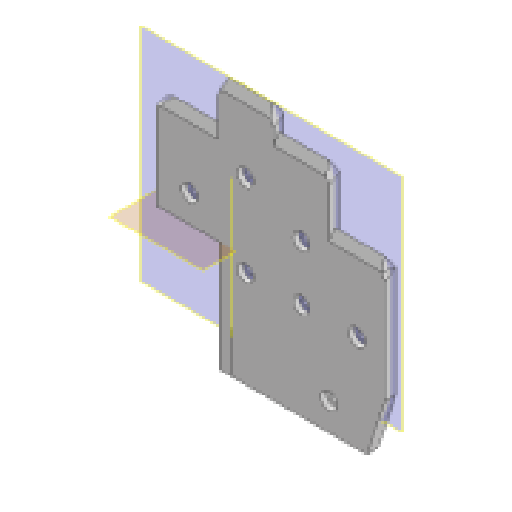
# Autodesk Inventor part: Palm
Saved by Autodesk Inventor 2025 (Build 290162010, 162A)
## iProperties
Created: 2024-12-07
Part Number: Palm
Material: Generic
Document SubType Name: Modeling
Designer: alexa
Density: 1 g/cm^3
Appearance: Default
Author: alexa
Autodesk Inventor part; units mm, degrees
ref_plane "YZ Plane" through (0, 0, 0) normal (1, 0, 0) x (0, 1, 0)
ref_plane "XZ Plane" through (0, 0, 0) normal (0, 1, 0) x (-1, 0, 0)
ref_plane "XY Plane" through (0, 0, 0) normal (0, 0, 1) x (1, 0, 0)
sketch "Sketch1" plane through (0, 0, 0) normal (0, 0, 1) x (1, 0, 0)
  line L0 (36.0199, -42.7926) -> (-34.4552, -42.7926)
  line L1 (-34.4552, -42.7926) -> (-34.4552, -11.0426)
  line L2 (-34.4552, -11.0426) -> (-73.3934, -11.0426)
  line L3 (-73.3934, -11.0426) -> (-73.3934, 18.523)
  line L4 (-73.3934, 18.523) -> (-69.4155, 29.59)
  line L5 (-69.4155, 29.59) -> (-40.9421, 29.59)
  line L6 (-40.9421, 29.59) -> (-40.9421, 49.91)
  line L7 (-40.9421, 49.91) -> (-15.2881, 49.91)
  line L8 (-15.2881, 49.91) -> (-15.2881, 39.75)
  line L9 (-15.2881, 39.75) -> (10.3659, 39.75)
  line L10 (10.3659, 39.75) -> (10.3659, 14.35)
  line L11 (10.3659, 14.35) -> (36.0199, 14.35)
  line L12 (36.0199, 14.35) -> (36.0199, -42.7926)
  point P0 (0, 0)
  dimension "d1" = 31.75
  dimension "d2" = 38.9382
  dimension "d3" = 29.5656
  dimension "d4" = 11.7602
  dimension "d5" = 19.77
  dimension "d6" = 28.4734
  dimension "d7" = 20.32
  dimension "d8" = 25.654
  dimension "d9" = 25.654
  dimension "d10" = 25.654
  dimension "d11" = 10.16
  dimension "d12" = 25.4
  constraints: 26 end point, 6 perpendicular, 3 horizontal, 3 vertical
  measures "d1" distance of L0.end L1.end
  measures "d2" distance of L1.end L2.end
  measures "d3" distance of L2.end L3.end
  measures "d4" distance of L3.end L4.end
  measures "d5" angle of L4 L1
  measures "d6" distance of L4.end L5.end
  measures "d7" distance of L5.end L6.end
  measures "d8" distance of L6.end L7.end
  measures "d9" distance of L8.end L9.end
  measures "d10" distance of L10.end L11.end
  measures "d11" distance of L7.end L8.end
  measures "d12" distance of L9.end L10.end
extrude "Extrusion1" add sketch "Sketch1" along normal blind 5.08
sketch "Sketch3" plane through (-34.4552, -42.7926, 0) normal (0, -1, 0) x (1, 0, 0)
  line L0 (0.0059, 0) -> (-3.82, 3.4008) projected
  line L1 (0, 0) -> (0, 5.08) projected
  line L2 (0, 0) -> (0, 5.08)
  line L3 (19.167, 5.08) -> (-6.487, 5.08) projected
  line L4 (0, 5.08) -> (0, 0)
  line L5 (0, 5.08) -> (-5.7091, 5.08)
  line L6 (-5.7091, 5.08) -> (0, 0)
  point P0 (34.4552, 0)
  point P1 (-5.7091, 5.08)
  point P2 (0, 0.0053)
  point P3 (-5.7091, 5.08)
  constraints: 8 end point, 2 point on line, 1 collinear, 1 perpendicular, 1 vertical
extrude "Extrusion3" add sketch "Sketch3" against normal blind 57.15
sketch "Sketch4" plane through (-73.3934, -11.0426, 0) normal (0, -1, 0) x (1, 0, 0)
  line L0 (17.1894, 19.3376) -> (-10.63, -11.9592) projected
  line L1 (0, 5.08) -> (38.9382, 5.08) projected
  line L2 (0, -0.0005) -> (0, 5.08)
  line L3 (0, 5.08) -> (4.516, 5.08)
  line L4 (4.516, 5.08) -> (0, -0.0005)
  point P0 (73.3934, 0)
  point P1 (33.2291, 5.08)
  point P2 (4.516, 5.08)
  constraints: 6 end point, 2 perpendicular, 2 point on line, 1 collinear
sketch "Sketch5" plane through (-40.9421, 29.59, 0) normal (-1, 0, 0) x (0, 0, 1)
  line L0 (2.54, 4.4068) -> (-12.7, -21.9897) projected
  line L1 (5.08, 0) -> (5.08, -11.067) projected
  line L2 (5.08, 0) -> (2.54, 4.4068)
  line L3 (2.54, 4.4068) -> (-0.0043, 0)
  line L4 (0, 0) -> (0, -11.067) projected
  line L5 (0, 0) -> (5.08, 0)
  line L6 (2.54, 4.4068) -> (0, 0)
  line L7 (0, 0) -> (5.08, 0)
  line L8 (5.08, 0) -> (2.54, 4.4068)
  point P0 (0, -29.59)
  constraints: 12 end point, 1 collinear, 1 horizontal, 1 perpendicular, 1 point on line
extrude "Extrusion4" add sketch "Sketch5" along normal up to surface surface through (-69.4155, 29.59, 0) normal (-0.941058, 0.3382452, 0)
extrude "Extrusion5" cut sketch "Sketch4" against normal blind 66.675
sketch "Sketch6" plane through (-40.9421, 29.59, 0) normal (0, 0.4993725, -0.8663874) x (-1, 0, 0)
  line L0 (25.654, 0.0178) -> (28.4749, 0.0064) projected
  line L1 (22.987, -32.5297) -> (22.987, 6.2121) projected
  line L2 (0, 5.0864) -> (26.8895, 5.0864) projected
  line L3 (22.987, 5.0864) -> (29.2176, 0.0225)
  line L4 (32.4508, -9.5873) -> (28.2515, 2.894) projected
  line L5 (29.2176, 0.0225) -> (22.987, 0.0225)
  line L6 (22.987, 0.0225) -> (22.987, 5.0864)
  line L7 (22.987, 5.0864) -> (26.8895, 5.0864)
  line L8 (26.8895, 5.0864) -> (28.2515, 2.894) projected
  line L9 (26.8895, 5.0864) -> (28.2515, 2.894)
  line L10 (28.2515, 2.894) -> (29.2176, 0.0225)
  point P0 (-40.9421, -25.6364)
  constraints: 12 end point, 4 point on line, 3 collinear, 1 horizontal, 1 perpendicular
extrude "Extrusion6" cut sketch "Sketch6" against normal blind 11.1125 contours L2 L8 L4 L3
sketch "Sketch7" plane through (-40.9421, 49.91, 0) normal (-1, 0, 0) x (0, 0, 1)
  line L0 (-12.7, -21.9897) -> (2.54, 4.4068) projected
  line L1 (0, 0) -> (5.08, 0) projected
  line L2 (2.54, 4.4068) -> (5.08, 0)
  line L3 (5.08, 0) -> (0, 0)
  line L4 (0, 0) -> (2.54, 4.4068)
  point P0 (0, -49.91)
  constraints: 6 end point, 1 collinear
extrude "Extrusion7" add sketch "Sketch7" against normal up to surface (25.654 mm away)
sketch "Sketch8" plane through (10.3659, 14.35, 0) normal (1, 0, 0) x (0, 0, -1)
  line L0 (12.7, -21.9897) -> (-2.54, 4.4068) projected
  line L1 (0, 0) -> (-5.08, 0) projected
  line L2 (-2.54, 4.4068) -> (-5.08, 0)
  line L3 (-5.08, 0) -> (0, 0.0074)
  line L4 (0, -25.3926) -> (0, 4.1741) projected
  line L5 (0, 0.0074) -> (-2.54, 4.4068)
  point P0 (0, -14.35)
  constraints: 6 end point, 2 point on line
extrude "Extrusion8" add sketch "Sketch8" along normal up to surface (25.654 mm away) contours L3 L2 L0
sketch "Sketch9" plane through (36.0199, 14.3574, 0) normal (0, 0.5, -0.8660254) x (-1, 0, 0)
  line L0 (2.667, -32.5754) -> (2.667, 6.1663) projected
  line L1 (2.54, 0) -> (0, 0) projected
  line L2 (0, 0) -> (2.667, 5.08)
  line L3 (25.654, 5.08) -> (0, 5.08) projected
  line L4 (0, 5.08) -> (0, 0) projected
  line L5 (2.667, 5.08) -> (0, 5.08)
  line L6 (0, 5.08) -> (0, 0)
  point P0 (36.0199, -12.4339)
  constraints: 6 end point, 2 perpendicular, 2 point on line
extrude "Extrusion9" cut sketch "Sketch9" against normal blind 14.2875
sketch "Sketch10" plane through (-15.2881, 39.75, 5.08) normal (1, 0, 0) x (0, 0, -1)
  line L0 (2.54, 4.4068) -> (17.78, -21.9897) projected
  line L1 (0, -25.4) -> (0, 0) projected
  line L2 (2.54, 4.4068) -> (0, 0)
  line L3 (0, 0) -> (5.08, 0)
  line L4 (5.08, 10.16) -> (5.08, -10.16) projected
  line L5 (5.08, 0) -> (0, 0)
  line L6 (5.08, 0) -> (2.54, 4.4068)
  point P0 (5.08, -39.75)
  constraints: 8 end point, 1 collinear, 1 midpoint
extrude "Extrusion10" add sketch "Sketch10" along normal up to surface (25.654 mm away) contours L6 L3 L2
sketch "Sketch11" plane through (10.3659, 39.75, 0) normal (0, 0.4993725, -0.8663874) x (-1, 0, 0)
  line L0 (2.667, -32.5297) -> (2.667, 6.2121) projected
  line L1 (2.54, 0.0178) -> (0, 0.0178) projected
  line L2 (0, -21.9999) -> (0, 0) projected
  line L3 (0, 0) -> (2.667, 5.0864)
  line L4 (25.654, 5.0864) -> (0, 5.0864) projected
  line L5 (2.667, 5.0864) -> (0, 5.0864)
  line L6 (0, 5.0864) -> (0, 0)
  point P0 (10.3659, -34.4389)
  constraints: 6 end point, 2 point on line, 1 collinear, 1 perpendicular
extrude "Extrusion11" cut sketch "Sketch11" against normal blind 14.2875
sketch "Sketch12" plane through (-15.2881, 49.91, 0) normal (0, 0.4993725, -0.8663874) x (-1, 0, 0)
  line L0 (2.667, -32.5297) -> (2.667, 6.2121) projected
  line L1 (2.54, 0.0178) -> (0, 0.0178) projected
  line L2 (22.987, -32.5297) -> (22.987, 6.2121) projected
  line L3 (23.114, 0.0178) -> (25.654, 0.0178) projected
  line L4 (0, 0.0178) -> (2.667, 5.0864)
  line L5 (25.654, 5.0864) -> (0, 5.0864) projected
  line L6 (2.667, 5.0864) -> (0, 5.0864)
  line L7 (0, 5.0864) -> (0, 0.0178)
  line L8 (25.654, 0.0178) -> (22.987, 5.0864)
  line L9 (22.987, 5.0864) -> (25.654, 5.0864)
  line L10 (25.654, 5.0864) -> (25.654, 0.0178)
  point P0 (-15.2881, -43.2414)
  point P1 (25.654, 5.0864)
  point P2 (22.987, 5.0864)
  constraints: 12 end point, 5 point on line, 2 perpendicular, 1 collinear
extrude "Extrusion12" cut sketch "Sketch12" against normal blind 30.1625
ref_plane "Work Plane1" through (-63.2227, -11.0426, -4.7625) normal (0, 1, 0) x (0, 0, -1)
sketch "Sketch13" plane through (0, 0, 5.08) normal (0, 0, 1) x (1, 0, 0)
  line L0 (-15.2881, 49.9174) -> (-15.2881, -36.4426) projected
  line L1 (-40.9421, 29.5974) -> (-40.9421, -36.4426) projected
  line L2 (-15.2881, 49.9174) -> (-15.2881, -36.4426) projected
  line L3 (10.3659, 39.7574) -> (10.3659, -36.4426) projected
  line L4 (36.0199, 14.3574) -> (36.0199, -36.4426) projected
  circle A0 centre (-28.1151, -17.3926) radius 1.778
  circle A1 centre (-2.4611, -17.3926) radius 1.778
  circle A2 centre (23.1929, -17.3926) radius 1.778
  line L5 (36.0199, -42.7926) -> (-40.1643, -42.7926) projected
  circle A3 centre (-28.1151, 20.7074) radius 1.778
  circle A4 centre (-2.4611, 8.0074) radius 1.778
  circle A5 centre (-53.7691, 1.6574) radius 1.778
  line L6 (-66.5961, 29.5974) -> (-66.5961, 14.3574) projected
  line L7 (-73.393, -11.0426) -> (-34.4552, -11.0426) projected
  point P0 (0, 0)
  dimension "d38" = 3.556
  dimension "d39" = 3.556
  dimension "d40" = 3.556
  dimension "d41" = 12.827
  dimension "d42" = 12.827
  dimension "d43" = 12.827
  dimension "d44" = 25.4
  dimension "d45" = 3.556
  dimension "d46" = 3.556
  dimension "d47" = 38.1
  dimension "d48" = 25.4
  dimension "d53" = 3.556
  dimension "d54" = 12.827
  dimension "d55" = 12.7
  constraints: 6 centre point, 2 horizontal alignment, 2 vertical alignment, 1 other
  measures "d38" diameter of A0
  measures "d39" diameter of A1
  measures "d40" diameter of A2
  measures "d41" distance from line of L0 A0.centre
  measures "d42" distance from line of L0 A1.centre
  measures "d43" distance from line of L3 A2.centre
  measures "d44" distance from line of L5 A0.centre
  measures "d45" diameter of A3
  measures "d46" diameter of A4
  measures "d47" distance of A3.centre A0.centre
  measures "d48" distance of A4.centre A1.centre
  measures "d53" diameter of A5
  measures "d54" distance from line of L1 A5.centre
extrude "Extrusion15" cut sketch "Sketch13" along normal blind 127 and the other way blind 127
ref_plane "Work Plane2" through (0, 0, 2.54) normal (0, 0, -1) x (-1, 0, 0)
sketch "Sketch17" plane through (0, 0, 2.54) normal (0, 0, -1) x (-1, 0, 0)
  circle A0 centre (28.1151, 20.7074) radius 1.778 projected
  circle A1 centre (28.1151, 20.7074) radius 3.81
  circle A2 centre (2.4611, 8.0074) radius 1.778 projected
  circle A3 centre (2.4611, 8.0074) radius 3.81
  circle A4 centre (2.4611, -17.3926) radius 1.778 projected
  circle A5 centre (2.4611, -17.3926) radius 3.81
  circle A6 centre (-23.1929, -17.3926) radius 1.778 projected
  circle A7 centre (-23.1929, -17.3926) radius 3.81
  circle A8 centre (28.1151, -17.3926) radius 1.778 projected
  circle A9 centre (28.1151, -17.3926) radius 3.81
  circle A10 centre (53.7691, 1.6574) radius 1.778 projected
  circle A11 centre (53.7691, 1.6574) radius 3.81
  point P0 (0, 0)
  dimension "d61" = 7.62
  dimension "d62" = 7.62
  dimension "d63" = 7.62
  dimension "d64" = 7.62
  dimension "d65" = 7.62
  dimension "d66" = 7.62
  constraints: 6 centre point, 6 coincident
  measures "d61" diameter of A11
  measures "d62" diameter of A1
  measures "d63" diameter of A3
  measures "d64" diameter of A9
  measures "d65" diameter of A5
  measures "d66" diameter of A7
extrude "Extrusion16" cut sketch "Sketch17" against normal blind 127 contours A1 | A3 | A4 | A5 | A6 | A7 | A9 | A11
sketch "Sketch18" plane through (0, 0, 5.08) normal (0, 0, 1) x (1, 0, 0)
  line L0 (-73.393, 14.3574) -> (-56.204, 14.3574) projected
  line L1 (-56.204, 14.3574) -> (-34.4493, 14.3574) projected
  line L2 (-34.4493, -36.4426) -> (-34.4493, 14.3574) projected
  line L3 (-68.8774, -11.0426) -> (-73.393, -11.0426) projected
  line L4 (-73.393, -11.0426) -> (-73.393, 18.5242) projected
  line L5 (-73.393, 14.3574) -> (-34.4552, 14.3574)
  line L6 (-34.4552, 14.3574) -> (-34.4552, -11.0426)
  line L7 (-73.393, -11.0426) -> (-73.393, 14.3574)
  line L8 (-73.393, -11.0426) -> (-34.4552, -11.0426) projected
  line L9 (-73.393, -11.0426) -> (-34.4552, -11.0426)
  point P0 (0, 0)
  constraints: 8 end point, 2 horizontal, 1 parallel, 1 perpendicular
extrude "Extrusion18" cut sketch "Sketch18" against normal blind 127
ref_plane "Work Plane3" through (-33.8301, -42.7926, 0) normal (1, 0, 0) x (0, 0, -1)
sketch "Sketch20" plane through (-33.8301, -42.7926, 0) normal (1, 0, 0) x (0, 0, -1)
  line L0 (-19.3376, 31.75) -> (0, 57.15) projected
  line L1 (-5.08, 57.15) -> (-5.08, 50.4774)
  line L2 (-5.08, 50.4774) -> (0, 57.15)
  line L3 (0, 0) -> (0, 57.1426) projected
  line L4 (0, 57.1426) -> (-5.08, 57.15)
  line L5 (-5.08, 50.4774) -> (-5.08, 31.75)
  line L6 (-5.08, 31.75) -> (-19.3376, 31.75)
  point P0 (0, 42.7926)
  point P1 (-0.0056, 57.1426)
  constraints: 10 end point, 1 perpendicular, 1 point on line, 1 vertical
extrude "Extrusion20" add sketch "Sketch20" against normal up to surface contours L1 L4 L0 surface through (-68.8774, -11.0426, 5.08) normal (0.7474093, 0, -0.6643638)
sketch "Sketch21" plane through (0, 0, 5.08) normal (0, 0, 1) x (1, 0, 0)
  line L0 (27.7649, -61.8426) -> (36.0199, -36.4426) projected
  line L1 (36.0199, -42.7926) -> (36.0199, 14.35) projected
  line L2 (36.0199, -36.4426) -> (36.0199, -42.7926)
  line L3 (36.0199, -42.7926) -> (33.9561, -42.7926)
  point P0 (0, 0)
  constraints: 4 end point, 1 collinear, 1 perpendicular, 1 point on line
extrude "Extrusion21" cut sketch "Sketch21" against normal blind 23.495
sketch "Sketch22" plane through (0, 0, 5.08) normal (0, 0, 1) x (1, 0, 0)
  line L0 (27.7649, -61.8426) -> (-34.4493, -61.8426) projected
  line L1 (27.7649, -61.8426) -> (36.0199, -36.4426) projected
  line L2 (-38.2751, -36.4426) -> (-38.2751, -61.8426) projected
  line L3 (-34.4493, -61.8426) -> (-48.4634, -61.8426) projected
  line L4 (33.9561, -42.7926) -> (-40.1643, -42.7926) projected
  line L5 (-34.4552, -42.7926) -> (-34.4552, -42.7926) projected
  line L6 (-34.4552, -42.7926) -> (-34.4493, -61.8426)
  point P0 (0, 0)
  point P1 (-38.2751, -42.7926)
  point P2 (-34.4552, 14.3574)
  constraints: 2 end point, 1 vertical alignment
extrude "Extrusion22" add sketch "Sketch22" against normal blind 5.08 contours L0 L6 L4 L1
sketch "Sketch23" plane through (-40.1643, -42.7926, 5.08) normal (0, -1, 0) x (1, 0, 0)
  line L0 (5.7091, -5.08) -> (5.7091, 0) projected
  line L1 (5.7091, 0) -> (0, 0) projected
  line L2 (0, 0) -> (5.7091, -5.08) projected
  point P0 (40.1643, -5.08)
extrude "Extrusion23" add sketch "Sketch23" along normal up to surface (19.05 mm away)
sketch "Sketch24" plane through (0, 0, 5.08) normal (0, 0, 1) x (1, 0, 0)
  line L0 (1.3489, -61.8426) -> (-6.2711, -61.8426) projected
  line L1 (27.0029, -61.8426) -> (19.3829, -61.8426) projected
  circle A0 centre (10.3659, -49.1426) radius 1.778
  line L2 (-34.4493, -61.8426) -> (27.7649, -61.8426) projected
  point P0 (0, 0)
  dimension "d84" = 3.556
  dimension "d85" = 18.034
  dimension "d86" = 9.017
  dimension "d87" = 12.7
  constraints: 1 centre point
  measures "d84" diameter of A0
  measures "d85" distance of L1.end L0.start
  measures "d86" horizontal distance of A0.centre L0.start
  measures "d87" distance from line of A0.centre L2
extrude "Extrusion24" cut sketch "Sketch24" against normal blind 33.3375
sketch "Sketch25" plane through (0, 0, 5.08) normal (0, 0, 1) x (1, 0, 0)
  circle A0 centre (10.3659, -49.1426) radius 1.778 projected
  circle A1 centre (10.3659, -49.1426) radius 3.81
  point P0 (0, 0)
  dimension "d90" = 7.62
  constraints: 1 centre point, 1 coincident
  measures "d90" diameter of A1
extrude "Extrusion25" cut sketch "Sketch25" against normal blind 2.54 contours A0 | A1
sketch "Sketch26" plane through (-40.1643, -11.0426, 5.08) normal (0, 1, 0) x (1, 0, 0)
  line L0 (5.7091, 0) -> (0, 0) projected
  line L1 (5.7091, 0) -> (5.7091, 5.08) projected
  line L2 (5.7091, 5.08) -> (0, 0) projected
  point P0 (40.1643, 5.08)
extrude "Extrusion26" add sketch "Sketch26" along normal up to next
equation "\"d45\" = d38"
equation "\"d46\" = d38"
equation "\"d62\" = d61"
equation "\"d63\" = d61"
equation "\"d64\" = d61"
equation "\"d65\" = d61"
equation "\"d66\" = d61"
equation "\"d86\" = 0.5 * d85"
body "Solid1"
